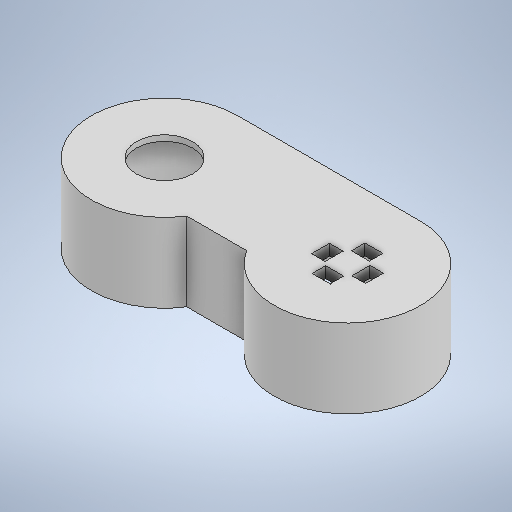
# Autodesk Inventor part: controller_v9_d1
Saved by Autodesk Inventor 2025.4 (Build 294407000, 407)
## iProperties
Created: 2026-07-26
Part Number: controller_v9_d1
Material: Generic
Document SubType Name: Modeling
Designer: Franchesca
Density: 1 g/cm^3
Appearance: Default
Author: Franchesca
Autodesk Inventor part; units mm, degrees
ref_plane "YZ Plane" through (0, 0, 0) normal (1, 0, 0) x (0, 1, 0)
ref_plane "XZ Plane" through (0, 0, 0) normal (0, 1, 0) x (-1, 0, 0)
ref_plane "XY Plane" through (0, 0, 0) normal (0, 0, 1) x (1, 0, 0)
sketch "Sketch1" plane through (0, 0, 0) normal (0, 1, 0) x (-1, 0, 0)
  circle A0 centre (0, 0) radius 30 construction
  circle A1 centre (0, 0) radius 32.5 construction
  line L0 (0, -30) -> (-81.4496, -30) construction
  circle A2 centre (-81.4496, 0) radius 30 construction
  circle A3 centre (-81.4496, 0) radius 32.5 construction
  line L1 (0, -32.5) -> (-81.4496, -32.5) construction
  line L2 (0, 32.5) -> (-81.4496, 32.5) construction
  line L3 (0, 30) -> (-81.4496, 30) construction
  line L4 (-40.7248, -32.5) -> (-40.7248, 32.5) construction
  line L5 (-40.7248, 30) -> (-40.7248, 14.2852) construction
  line L6 (-81.4496, -30) -> (-81.4496, 30) construction
  line L7 (-40.7248, 14.2852) -> (-40.7248, 16.7852) construction
  arc A4 (0, -30) -> (30, 0) centre (0, 0) ccw
  arc A5 (30, 0) -> (0, 30) centre (0, 0) ccw
  arc A6 (-111.4496, 0) -> (-81.4496, -30) centre (-81.4496, 0) ccw
  arc A7 (-81.4496, 30) -> (-111.4496, 0) centre (-81.4496, 0) ccw
  arc A8 (0, -32.5) -> (32.5, 0) centre (0, 0) ccw
  arc A9 (32.5, 0) -> (0, 32.5) centre (0, 0) ccw
  arc A10 (-81.4496, 32.5) -> (-113.9496, 0) centre (-81.4496, 0) ccw
  arc A11 (-113.9496, 0) -> (-81.4496, -32.5) centre (-81.4496, 0) ccw
  line L8 (0, -30) -> (-81.4496, -30)
  line L9 (0, -32.5) -> (-81.4496, -32.5)
  line L10 (-40.7248, -30) -> (-40.7248, 15) construction
  line L11 (-40.7248, 15) -> (-28.8314, 15) construction
  line L12 (-40.7248, 15) -> (-52.6182, 15) construction
  line L13 (-40.7248, 15) -> (-40.7248, 17.5) construction
  line L14 (-40.7248, 17.5) -> (-27.3861, 17.5)
  line L15 (-40.7248, 17.5) -> (-54.0635, 17.5)
  line L16 (-52.6182, 15) -> (-55.4688, 15) construction
  line L17 (-28.8314, 15) -> (-25.9836, 15) construction
  arc A12 (0, 30) -> (-25.9836, 14.9951) centre (0, 0) ccw
  arc A13 (-55.4688, 15) -> (-81.4496, 30) centre (-81.4496, 0) ccw
  line L18 (-25.9836, 14.9951) -> (-55.4688, 15)
  arc A14 (0, 32.5) -> (-27.3861, 17.5) centre (0, 0) ccw
  arc A15 (-54.0635, 17.5) -> (-81.4496, 32.5) centre (-81.4496, 0) ccw
  circle A16 centre (0, 0) radius 12.5
  line L19 (-81.4496, 0) -> (-81.4496, -4.25) construction
  line L20 (-81.4496, 0) -> (-81.4496, 4.25) construction
  line L21 (-81.4496, 0) -> (-77.1996, 0) construction
  line L22 (-81.4496, 0) -> (-85.6996, 0) construction
  line L23 (-77.1996, 0) -> (-77.1996, -4.25)
  line L24 (-77.1996, -4.25) -> (-85.6996, -4.25)
  line L25 (-85.6996, -4.25) -> (-85.6996, 4.25)
  line L26 (-85.6996, 4.25) -> (-77.1996, 4.25)
  line L27 (-77.1996, 4.25) -> (-77.1996, 0)
  line L28 (-81.4496, -4.25) -> (-81.4496, -5.75) construction
  line L29 (-85.6996, 0) -> (-87.1996, 0) construction
  line L30 (-81.4496, 4.25) -> (-81.4496, 5.75) construction
  line L31 (-77.1996, 0) -> (-75.6996, 0) construction
  line L32 (-77.1996, 4.25) -> (-75.6996, 4.25) construction
  line L33 (-75.6996, 4.25) -> (-75.6996, -3.75)
  line L34 (-75.6996, -3.75) -> (-69.6996, -3.75)
  line L35 (-69.6996, -3.75) -> (-69.6996, 4.25)
  line L36 (-69.6996, 4.25) -> (-75.6996, 4.25)
  line L37 (-87.1996, -4.25) -> (-87.1996, 3.75)
  line L38 (-87.1996, 3.75) -> (-93.1996, 3.75)
  line L39 (-93.1996, 3.75) -> (-93.1996, -4.25)
  line L40 (-93.1996, -4.25) -> (-87.1996, -4.25)
  line L41 (-81.4496, -5.75) -> (-77.4496, -5.75)
  line L42 (-81.4496, -5.75) -> (-85.4496, -5.75)
  line L43 (-85.4496, -5.75) -> (-85.4496, -11.75)
  line L44 (-85.4496, -11.75) -> (-77.4496, -11.75)
  line L45 (-77.4496, -11.75) -> (-77.4496, -5.75)
  line L46 (-81.4496, 5.75) -> (-77.4496, 5.75)
  line L47 (-81.4496, 5.75) -> (-85.4496, 5.75)
  line L48 (-85.4496, 5.75) -> (-85.4496, 11.75)
  line L49 (-85.4496, 11.75) -> (-77.4496, 11.75)
  line L50 (-77.4496, 11.75) -> (-77.4496, 5.75)
  line L51 (0, 0) -> (-16, 0) construction
  line L52 (0, 0) -> (-15, 0) construction
  line L53 (0, 0) -> (-14, 0) construction
  line L54 (0, 12.5) -> (-16, 12.5) construction
  line L55 (0, -12.5) -> (-16, -12.5) construction
  line L56 (-15, 0) -> (-15, 12.5) construction
  line L57 (-15, 0) -> (-15, -12.5) construction
  line L58 (-14, 0) -> (-14, -12.5) construction
  line L59 (-14, 0) -> (-14, 12.5) construction
  line L60 (-16, 12.5) -> (-16, 0) construction
  line L61 (-16, 0) -> (-16, -12.5) construction
  line L62 (-16, -12.5) -> (-16, -8.5) construction
  line L63 (-16, 12.5) -> (-16, 8.5) construction
  line L64 (-14, -12.5) -> (-14, -8.5) construction
  line L65 (-14, 12.5) -> (-14, 8.5) construction
  line L66 (-14, -8.5) -> (-33, -8.5)
  line L67 (-14, 8.5) -> (-14, -8.5)
  line L68 (-14, -12.5) -> (-14, -7.5) construction
  line L69 (-14, 12.5) -> (-14, 7.5) construction
  line L70 (-15, -7.5) -> (-15, 7.5)
  line L71 (-14, 8.5) -> (-33, 8.5)
  line L72 (-33, 7.5) -> (-33, 8.5)
  line L73 (-15, 7.5) -> (-33, 7.5)
  line L74 (-15, -7.5) -> (-33, -7.5)
  line L75 (-33, -7.5) -> (-33, -8.5)
  line L76 (-33, -7.5) -> (-33, 7.5)
  line L77 (0, -12.5) -> (0, -15.5) construction
  line L78 (0, 12.5) -> (0, 15.5) construction
  line L79 (12.5, 0) -> (15.5, 0) construction
  line L80 (15.5, 0) -> (15.5, -15.5)
  line L81 (15.5, -15.5) -> (0, -15.5)
  line L82 (0, 15.5) -> (15.5, 15.5)
  line L83 (15.5, 15.5) -> (15.5, 0)
  line L84 (-33, 0) -> (-36, 0) construction
  line L85 (-36, 0) -> (-36, -15.5)
  line L86 (-36, -15.5) -> (0, -15.5)
  line L87 (15.5, 15.5) -> (-25.6856, 15.5)
  line L88 (-36, 0) -> (-36, 14.9967)
  point P0 (-81.4496, -4.25)
  point P1 (-79.4496, 5.75)
  dimension "d0" = 60
  dimension "d1" = 65
  dimension "d2" = 81.4496
  dimension "d3" = 60
  dimension "d4" = 65
  dimension "d7" = 2.5
  dimension "d10" = 2.5
  dimension "d12" = 25
  dimension "d13" = 81.4496
  dimension "d14" = 2.5
  dimension "d15" = 4.25
  dimension "d16" = 4.25
  dimension "d17" = 4.25
  dimension "d18" = 4.25
  dimension "d21" = 1.5
  dimension "d23" = 8
  dimension "d24" = 6
  dimension "d25" = 50
  dimension "d26" = 45
  dimension "d27" = 25.75
  dimension "d28" = 25.75
  dimension "d29" = 8
  dimension "d30" = 6
  dimension "d32" = 4
  dimension "d33" = 4
  dimension "d34" = 6
  dimension "d35" = 4
  dimension "d36" = 4
  dimension "d37" = 6
  dimension "d38" = 1.5
  dimension "d40" = 1.5
  dimension "d41" = 1.5
  dimension "d42" = 1.5
  dimension "d43" = 8
  dimension "d44" = 16
  dimension "d45" = 15
  dimension "d46" = 14
  dimension "d49" = 4
  dimension "d50" = 4
  dimension "d51" = 19
  dimension "d53" = 5
  dimension "d54" = 5
  dimension "d55" = 19
  dimension "d56" = 18
  dimension "d57" = 18
  dimension "d58" = 15
  dimension "d59" = 3
  dimension "d60" = 3
  dimension "d61" = 3
  dimension "d62" = 3
  constraints: 178 end point, 46 point on circle, 30 point on line, 27 perpendicular, 18 horizontal, 17 centre point, 10 concentric, 10 tangent, 7 midpoint, 5 parallel, 4 coincident, 4 collinear, 4 vertical
  measures "d0" diameter of A0
  measures "d1" diameter of A1
  measures "d2" distance of L0.start L0.end
  measures "d3" diameter of A2
  measures "d4" diameter of A3
  measures "d7" distance between parallel lines of L0 L1
  measures "d10" distance of L10.end L13.end
  measures "d12" diameter of A16
  measures "d13" distance of L1.start L1.end
  measures "d14" radial gap between concentric circles of A2 A3
  measures "d15" distance of L19.start L19.end
  measures "d16" distance of L19.start L20.end
  measures "d17" distance of L19.start L21.end
  measures "d18" distance of L19.start L22.end
  measures "d21" distance of L20.end L30.end
  measures "d23" distance of L32.end L33.end
  measures "d24" distance of L33.end L34.end
  measures "d25" distance between parallel lines of L14 L9
  measures "d26" distance between parallel lines of L0 L11
  measures "d27" distance from line of L3.end L26
  measures "d28" distance of L0.end point (-81.45, -4.25)
  measures "d29" distance of L37.start L37.end
  measures "d30" distance of L37.end L38.end
  measures "d32" distance of L28.end L41.end
  measures "d33" distance of L28.end L42.end
  measures "d34" distance of L42.end L43.end
  measures "d35" distance of L30.end L46.end
  measures "d36" distance of L30.end L47.end
  measures "d37" distance of L47.end L48.end
  measures "d38" distance between parallel lines of L23 L33
  measures "d40" distance between parallel lines of L37 L25
  measures "d41" distance between parallel lines of L24 L42
  measures "d42" distance from line of point (-79.45, 5.75) L26
  measures "d43" distance between parallel lines of L48 L50
  measures "d44" distance of L51.start L51.end
  measures "d45" distance of L51.start L52.end
  measures "d46" distance of L51.start L53.end
  measures "d49" distance of L58.end L64.end
  measures "d50" distance of L59.end L65.end
  measures "d51" distance of L64.end L66.end
  measures "d53" distance of L58.end L68.end
  measures "d54" distance of L59.end L69.end
  measures "d55" distance of L65.end L71.end
  measures "d56" distance of L70.end L72.start
  measures "d57" distance of L70.start L74.end
  measures "d58" distance between parallel lines of L73 L74
  measures "d59" distance of L55.start L77.end
  measures "d60" distance of L54.start L78.end
  measures "d61" distance of L79.start L79.end
  measures "d62" distance of L84.start L84.end
extrude "Extrusion1" add sketch "Sketch1" against normal blind 35 contours L9 A11 A10 A15 L15 L14 A14 A9 A8
extrude "Extrusion2" add sketch "Sketch1" against normal blind 2.5 contours L87 L82 L83 L80 L81 L86 L85 L88 L18 A12
extrude "Extrusion3" add sketch "Sketch1" against normal blind 4 contours L76 L73 L70 L74
extrude "Extrusion4" add sketch "Sketch1" against normal blind 20 contours L66 L75 L74 L70 L73 L72 L71 L67
extrude "Extrusion5" add sketch "Sketch1" against normal blind 5 contours L8 A6 A7 A13 L18 L88 L85 L86 L81 L80 L83 L82 L87 A12 A5 A4
extrude "Extrusion6" add sketch "Sketch1" against normal blind 1 contours L23 L24 L25 L26 L27
body "Solid1"
